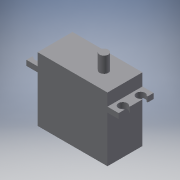
# Autodesk Inventor part: 馬達
Saved by Autodesk Inventor 2016 (Build 200138000, 138)
## iProperties
Created: 2017-12-26
Part Number: 馬達
Material: 一般
Document SubType Name: Modeling
Designer: user
Density: 1 g/cm^3
Appearance: 預設
Author: user
Autodesk Inventor part; units mm, degrees
ref_plane "YZ Plane" through (0, 0, 0) normal (1, 0, 0) x (0, 1, 0)
ref_plane "XZ Plane" through (0, 0, 0) normal (0, 1, 0) x (-1, 0, 0)
ref_plane "XY Plane" through (0, 0, 0) normal (0, 0, 1) x (1, 0, 0)
sketch "草圖1" plane through (0, 0, 0) normal (0, 1, 0) x (-1, 0, 0)
  line L0 (20, -18.25) -> (-20, -18.25)
  line L1 (-20, -18.25) -> (-20, 18.25)
  line L2 (-20, 18.25) -> (20, 18.25)
  line L3 (20, 18.25) -> (20, -18.25)
  line L4 (20, -18.25) -> (-20, 18.25) construction
  line L5 (-20, -18.25) -> (20, 18.25) construction
  line L6 (26.4, 11.25) -> (-26.4, 11.25)
  line L7 (-26.4, 11.25) -> (-26.4, 8.25)
  line L8 (-26.4, 8.25) -> (26.4, 8.25)
  line L9 (26.4, 8.25) -> (26.4, 11.25)
  point P0 (0, 0)
  point P1 (0, 11.25)
  point P2 (0, 18.25)
  dimension "d0" = 40
  dimension "d1" = 36.5
  dimension "d2" = 3
  dimension "d4" = 52.8
  dimension "d5" = 26.5
  constraints: 20 end point, 4 midpoint, 4 parallel, 2 horizontal, 2 perpendicular, 1 vertical alignment
  measures "d0" distance of L0.start L0.end
  measures "d1" distance of L0.end L1.end
  measures "d2" distance of L6.end L7.end
  measures "d4" distance of L7.end L8.end
  measures "d5" distance between parallel lines of L8 L0
extrude "擠出1" add sketch "草圖1" along normal mid plane 20
sketch "草圖2" plane through (20, -10, 11.25) normal (0, 0, 1) x (1, 0, 0)
  line L0 (-40, 0) -> (-40, 20) construction
  line L1 (0, 20) -> (-40, 20) construction
  line L2 (0, 20) -> (0, 0) construction
  line L3 (-40, 0) -> (0, 0) construction
  line L4 (-43.9, 4.9) -> (3.9, 4.9) construction
  line L5 (3.9, 4.9) -> (3.9, 15.1) construction
  line L6 (3.9, 15.1) -> (-43.9, 15.1) construction
  line L7 (-43.9, 15.1) -> (-43.9, 4.9) construction
  line L8 (-43.9, 4.9) -> (3.9, 15.1) construction
  line L9 (3.9, 4.9) -> (-43.9, 15.1) construction
  point P0 (-20, 10)
  dimension "d8" = 47.8
  dimension "d9" = 10.2
  constraints: 12 end point, 4 coincident, 2 midpoint, 2 parallel, 1 horizontal, 1 perpendicular
  measures "d8" distance of L5.end L6.end
  measures "d9" distance of L4.end L5.end
hole "孔1" at (23.9, 5.1, 11.25) at (23.9, -5.1, 11.25) at (-23.9, -5.1, 11.25) at (-23.9, 5.1, 11.25) direction (0, 0, -1) diameter 5 depth 8 tip angle 118
sketch "草圖3" plane through (20, -10, 11.25) normal (0, 0, 1) x (1, 0, 0)
  circle A0 centre (3.9, 15.1) radius 2.5 construction
  line L0 (3.9, 16.6) -> (13.7017, 16.6)
  line L1 (13.7017, 16.6) -> (13.7017, 13.6)
  line L2 (13.7017, 13.6) -> (3.9, 13.6)
  line L3 (3.9, 13.6) -> (3.9, 16.6)
  point P0 (-20, 10)
  point P1 (6.4, 15.1)
  dimension "d17" = 3
  constraints: 8 end point, 2 parallel, 1 coincident, 1 horizontal, 1 horizontal alignment, 1 midpoint, 1 perpendicular
  measures "d17" distance of L0.end L1.end
extrude "擠出2" cut sketch "草圖3" against normal blind 20
mirror "鏡射1" about plane through (0, 0, 0) normal (0, 1, 0) of "擠出2"
mirror "鏡射2" about plane through (0, 0, 0) normal (1, 0, 0) of "擠出2", "鏡射1"
sketch "草圖4" plane through (-20, 10, 18.25) normal (0, 0, 1) x (1, 0, 0)
  circle A0 centre (28, -10) radius 2.5
  line L0 (40, 0) -> (40, -20) construction
  line L1 (0, 0) -> (0, -20) projected
  point P0 (20, -10)
  dimension "d20" = 5
  dimension "d25" = 12
  constraints: 1 centre point, 1 horizontal alignment
  measures "d20" diameter of A0
  measures "d25" distance from line of L0 A0.centre
extrude "擠出3" add sketch "草圖4" along normal blind 9
